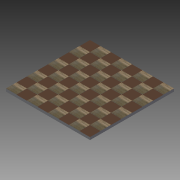
# Autodesk Inventor part: Board 001
Saved by Autodesk Inventor 2015 SP1 (Build 190203100, 203)
## iProperties
Created: 2015-06-07
Part Number: Board 001
Material: Generic
Document SubType Name: Modeling
Designer: Nathan
Density: 1 g/cm^3
Appearance: Default
Author: Nathan
Autodesk Inventor part; units mm, degrees
ref_plane "YZ Plane" through (0, 0, 0) normal (1, 0, 0) x (0, 1, 0)
ref_plane "XZ Plane" through (0, 0, 0) normal (0, 1, 0) x (-1, 0, 0)
ref_plane "XY Plane" through (0, 0, 0) normal (0, 0, 1) x (1, 0, 0)
sketch "Sketch1" plane through (0, 0, 0) normal (0, 1, 0) x (-1, 0, 0)
  line L0 (-180, 180) -> (180, 180)
  line L1 (180, 180) -> (180, -180)
  line L2 (180, -180) -> (-180, -180)
  line L3 (-180, -180) -> (-180, 180)
  line L4 (-180, 180) -> (180, -180) construction
  line L5 (180, 180) -> (-180, -180) construction
  line L6 (180, 180) -> (135, 180)
  line L7 (135, 180) -> (135, 135)
  line L8 (135, 135) -> (180, 135)
  line L9 (180, 135) -> (180, 180)
  line L10 (180, 135) -> (135, 135)
  line L11 (135, 135) -> (135, 90)
  line L12 (135, 90) -> (180, 90)
  line L13 (180, 90) -> (180, 135)
  line L14 (180, 90) -> (135, 90)
  line L15 (135, 90) -> (135, 45)
  line L16 (135, 45) -> (180, 45)
  line L17 (180, 45) -> (180, 90)
  line L18 (180, 45) -> (135, 45)
  line L19 (135, 45) -> (135, 0)
  line L20 (135, 0) -> (180, 0)
  line L21 (180, 0) -> (180, 45)
  line L22 (180, 0) -> (135, 0)
  line L23 (135, 0) -> (135, -45)
  line L24 (135, -45) -> (180, -45)
  line L25 (180, -45) -> (180, 0)
  line L26 (180, -45) -> (135, -45)
  line L27 (135, -45) -> (135, -90)
  line L28 (135, -90) -> (180, -90)
  line L29 (180, -90) -> (180, -45)
  line L30 (180, -90) -> (135, -90)
  line L31 (135, -90) -> (135, -135)
  line L32 (135, -135) -> (180, -135)
  line L33 (180, -135) -> (180, -90)
  line L34 (180, -135) -> (135, -135)
  line L35 (135, -135) -> (135, -180)
  line L36 (135, -180) -> (180, -180)
  line L37 (180, -180) -> (180, -135)
  line L38 (135, 180) -> (90, 180)
  line L39 (90, 180) -> (90, 135)
  line L40 (90, 135) -> (135, 135)
  line L41 (135, 135) -> (135, 180)
  line L42 (135, 135) -> (90, 135)
  line L43 (90, 135) -> (90, 90)
  line L44 (90, 90) -> (135, 90)
  line L45 (135, 90) -> (135, 135)
  line L46 (135, 90) -> (90, 90)
  line L47 (90, 90) -> (90, 45)
  line L48 (90, 45) -> (135, 45)
  line L49 (135, 45) -> (135, 90)
  line L50 (135, 45) -> (90, 45)
  line L51 (90, 45) -> (90, 0)
  line L52 (90, 0) -> (135, 0)
  line L53 (135, 0) -> (135, 45)
  line L54 (135, 0) -> (90, 0)
  line L55 (90, 0) -> (90, -45)
  line L56 (90, -45) -> (135, -45)
  line L57 (135, -45) -> (135, 0)
  line L58 (135, -45) -> (90, -45)
  line L59 (90, -45) -> (90, -90)
  line L60 (90, -90) -> (135, -90)
  line L61 (135, -90) -> (135, -45)
  line L62 (135, -90) -> (90, -90)
  line L63 (90, -90) -> (90, -135)
  line L64 (90, -135) -> (135, -135)
  line L65 (135, -135) -> (135, -90)
  line L66 (135, -135) -> (90, -135)
  line L67 (90, -135) -> (90, -180)
  line L68 (90, -180) -> (135, -180)
  line L69 (135, -180) -> (135, -135)
  line L70 (90, 180) -> (45, 180)
  line L71 (45, 180) -> (45, 135)
  line L72 (45, 135) -> (90, 135)
  line L73 (90, 135) -> (90, 180)
  line L74 (90, 135) -> (45, 135)
  line L75 (45, 135) -> (45, 90)
  line L76 (45, 90) -> (90, 90)
  line L77 (90, 90) -> (90, 135)
  line L78 (90, 90) -> (45, 90)
  line L79 (45, 90) -> (45, 45)
  line L80 (45, 45) -> (90, 45)
  line L81 (90, 45) -> (90, 90)
  line L82 (90, 45) -> (45, 45)
  line L83 (45, 45) -> (45, 0)
  line L84 (45, 0) -> (90, 0)
  line L85 (90, 0) -> (90, 45)
  line L86 (90, 0) -> (45, 0)
  line L87 (45, 0) -> (45, -45)
  line L88 (45, -45) -> (90, -45)
  line L89 (90, -45) -> (90, 0)
  line L90 (90, -45) -> (45, -45)
  line L91 (45, -45) -> (45, -90)
  line L92 (45, -90) -> (90, -90)
  line L93 (90, -90) -> (90, -45)
  line L94 (90, -90) -> (45, -90)
  line L95 (45, -90) -> (45, -135)
  line L96 (45, -135) -> (90, -135)
  line L97 (90, -135) -> (90, -90)
  line L98 (90, -135) -> (45, -135)
  line L99 (45, -135) -> (45, -180)
  line L100 (45, -180) -> (90, -180)
  line L101 (90, -180) -> (90, -135)
  line L102 (45, 180) -> (0, 180)
  line L103 (0, 180) -> (0, 135)
  line L104 (0, 135) -> (45, 135)
  line L105 (45, 135) -> (45, 180)
  line L106 (45, 135) -> (0, 135)
  line L107 (0, 135) -> (0, 90)
  line L108 (0, 90) -> (45, 90)
  line L109 (45, 90) -> (45, 135)
  line L110 (45, 90) -> (0, 90)
  line L111 (0, 90) -> (0, 45)
  line L112 (0, 45) -> (45, 45)
  line L113 (45, 45) -> (45, 90)
  line L114 (45, 45) -> (0, 45)
  line L115 (0, 45) -> (0, 0)
  line L116 (0, 0) -> (45, 0)
  line L117 (45, 0) -> (45, 45)
  line L118 (45, 0) -> (0, 0)
  line L119 (0, 0) -> (0, -45)
  line L120 (0, -45) -> (45, -45)
  line L121 (45, -45) -> (45, 0)
  line L122 (45, -45) -> (0, -45)
  line L123 (0, -45) -> (0, -90)
  line L124 (0, -90) -> (45, -90)
  line L125 (45, -90) -> (45, -45)
  line L126 (45, -90) -> (0, -90)
  line L127 (0, -90) -> (0, -135)
  line L128 (0, -135) -> (45, -135)
  line L129 (45, -135) -> (45, -90)
  line L130 (45, -135) -> (0, -135)
  line L131 (0, -135) -> (0, -180)
  line L132 (0, -180) -> (45, -180)
  line L133 (45, -180) -> (45, -135)
  line L134 (0, 180) -> (-45, 180)
  line L135 (-45, 180) -> (-45, 135)
  line L136 (-45, 135) -> (0, 135)
  line L137 (0, 135) -> (0, 180)
  line L138 (0, 135) -> (-45, 135)
  line L139 (-45, 135) -> (-45, 90)
  line L140 (-45, 90) -> (0, 90)
  line L141 (0, 90) -> (0, 135)
  line L142 (0, 90) -> (-45, 90)
  line L143 (-45, 90) -> (-45, 45)
  line L144 (-45, 45) -> (0, 45)
  line L145 (0, 45) -> (0, 90)
  line L146 (0, 45) -> (-45, 45)
  line L147 (-45, 45) -> (-45, 0)
  line L148 (-45, 0) -> (0, 0)
  line L149 (0, 0) -> (0, 45)
  line L150 (0, 0) -> (-45, 0)
  line L151 (-45, 0) -> (-45, -45)
  line L152 (-45, -45) -> (0, -45)
  line L153 (0, -45) -> (0, 0)
  line L154 (0, -45) -> (-45, -45)
  line L155 (-45, -45) -> (-45, -90)
  line L156 (-45, -90) -> (0, -90)
  line L157 (0, -90) -> (0, -45)
  line L158 (0, -90) -> (-45, -90)
  line L159 (-45, -90) -> (-45, -135)
  line L160 (-45, -135) -> (0, -135)
  line L161 (0, -135) -> (0, -90)
  line L162 (0, -135) -> (-45, -135)
  line L163 (-45, -135) -> (-45, -180)
  line L164 (-45, -180) -> (0, -180)
  line L165 (0, -180) -> (0, -135)
  line L166 (-45, 180) -> (-90, 180)
  line L167 (-90, 180) -> (-90, 135)
  line L168 (-90, 135) -> (-45, 135)
  line L169 (-45, 135) -> (-45, 180)
  line L170 (-45, 135) -> (-90, 135)
  line L171 (-90, 135) -> (-90, 90)
  line L172 (-90, 90) -> (-45, 90)
  line L173 (-45, 90) -> (-45, 135)
  line L174 (-45, 90) -> (-90, 90)
  line L175 (-90, 90) -> (-90, 45)
  line L176 (-90, 45) -> (-45, 45)
  line L177 (-45, 45) -> (-45, 90)
  line L178 (-45, 45) -> (-90, 45)
  line L179 (-90, 45) -> (-90, 0)
  line L180 (-90, 0) -> (-45, 0)
  line L181 (-45, 0) -> (-45, 45)
  line L182 (-45, 0) -> (-90, 0)
  line L183 (-90, 0) -> (-90, -45)
  line L184 (-90, -45) -> (-45, -45)
  line L185 (-45, -45) -> (-45, 0)
  line L186 (-45, -45) -> (-90, -45)
  line L187 (-90, -45) -> (-90, -90)
  line L188 (-90, -90) -> (-45, -90)
  line L189 (-45, -90) -> (-45, -45)
  line L190 (-45, -90) -> (-90, -90)
  line L191 (-90, -90) -> (-90, -135)
  line L192 (-90, -135) -> (-45, -135)
  line L193 (-45, -135) -> (-45, -90)
  line L194 (-45, -135) -> (-90, -135)
  line L195 (-90, -135) -> (-90, -180)
  line L196 (-90, -180) -> (-45, -180)
  line L197 (-45, -180) -> (-45, -135)
  line L198 (-90, 180) -> (-135, 180)
  line L199 (-135, 180) -> (-135, 135)
  line L200 (-135, 135) -> (-90, 135)
  line L201 (-90, 135) -> (-90, 180)
  line L202 (-90, 135) -> (-135, 135)
  line L203 (-135, 135) -> (-135, 90)
  line L204 (-135, 90) -> (-90, 90)
  line L205 (-90, 90) -> (-90, 135)
  line L206 (-90, 90) -> (-135, 90)
  line L207 (-135, 90) -> (-135, 45)
  line L208 (-135, 45) -> (-90, 45)
  line L209 (-90, 45) -> (-90, 90)
  line L210 (-90, 45) -> (-135, 45)
  line L211 (-135, 45) -> (-135, 0)
  line L212 (-135, 0) -> (-90, 0)
  line L213 (-90, 0) -> (-90, 45)
  line L214 (-90, 0) -> (-135, 0)
  line L215 (-135, 0) -> (-135, -45)
  line L216 (-135, -45) -> (-90, -45)
  line L217 (-90, -45) -> (-90, 0)
  line L218 (-90, -45) -> (-135, -45)
  line L219 (-135, -45) -> (-135, -90)
  line L220 (-135, -90) -> (-90, -90)
  line L221 (-90, -90) -> (-90, -45)
  line L222 (-90, -90) -> (-135, -90)
  line L223 (-135, -90) -> (-135, -135)
  line L224 (-135, -135) -> (-90, -135)
  line L225 (-90, -135) -> (-90, -90)
  line L226 (-90, -135) -> (-135, -135)
  line L227 (-135, -135) -> (-135, -180)
  line L228 (-135, -180) -> (-90, -180)
  line L229 (-90, -180) -> (-90, -135)
  line L230 (-135, 180) -> (-180, 180)
  line L231 (-180, 180) -> (-180, 135)
  line L232 (-180, 135) -> (-135, 135)
  line L233 (-135, 135) -> (-135, 180)
  line L234 (-135, 135) -> (-180, 135)
  line L235 (-180, 135) -> (-180, 90)
  line L236 (-180, 90) -> (-135, 90)
  line L237 (-135, 90) -> (-135, 135)
  line L238 (-135, 90) -> (-180, 90)
  line L239 (-180, 90) -> (-180, 45)
  line L240 (-180, 45) -> (-135, 45)
  line L241 (-135, 45) -> (-135, 90)
  line L242 (-135, 45) -> (-180, 45)
  line L243 (-180, 45) -> (-180, 0)
  line L244 (-180, 0) -> (-135, 0)
  line L245 (-135, 0) -> (-135, 45)
  line L246 (-135, 0) -> (-180, 0)
  line L247 (-180, 0) -> (-180, -45)
  line L248 (-180, -45) -> (-135, -45)
  line L249 (-135, -45) -> (-135, 0)
  line L250 (-135, -45) -> (-180, -45)
  line L251 (-180, -45) -> (-180, -90)
  line L252 (-180, -90) -> (-135, -90)
  line L253 (-135, -90) -> (-135, -45)
  line L254 (-135, -90) -> (-180, -90)
  line L255 (-180, -90) -> (-180, -135)
  line L256 (-180, -135) -> (-135, -135)
  line L257 (-135, -135) -> (-135, -90)
  line L258 (-135, -135) -> (-180, -135)
  line L259 (-180, -135) -> (-180, -180)
  line L260 (-180, -180) -> (-135, -180)
  line L261 (-135, -180) -> (-135, -135)
  dimension "d0" = 360
  dimension "d1" = 360
  dimension "d2" = 45
  dimension "d3" = 45
  dimension "d6" = 45
  dimension "d9" = 45
  constraints: 524 end point, 4 parallel, 3 horizontal, 2 midpoint, 2 perpendicular, 1 vertical, 504 other
  measures "d0" distance of L1.end L2.end
  measures "d1" distance of L0.end L1.end
  measures "d2" distance of L8.end L7.end
  measures "d3" distance of L7.end L6.end
  measures "d6" distance of L0.end L10.start
  measures "d9" distance of L0.end L38.start
extrude "Extrusion1" add sketch "Sketch1" against normal blind 11
sketch "Sketch2" plane through (0, 0, 0) normal (0, 1, 0) x (1, 0, 0)
  line L0 (-180, -180) -> (-135, -180)
  line L1 (-135, -180) -> (-135, -135)
  line L2 (-135, -135) -> (-180, -135)
  line L3 (-180, -135) -> (-180, -180)
  line L4 (-180, -90) -> (-135, -90)
  line L5 (-135, -90) -> (-135, -45)
  line L6 (-135, -45) -> (-180, -45)
  line L7 (-180, -45) -> (-180, -90)
  line L8 (-180, 0) -> (-135, 0)
  line L9 (-135, 0) -> (-135, 45)
  line L10 (-135, 45) -> (-180, 45)
  line L11 (-180, 45) -> (-180, 0)
  line L12 (-180, 90) -> (-135, 90)
  line L13 (-135, 90) -> (-135, 135)
  line L14 (-135, 135) -> (-180, 135)
  line L15 (-180, 135) -> (-180, 90)
  line L16 (-90, -180) -> (-45, -180)
  line L17 (-45, -180) -> (-45, -135)
  line L18 (-45, -135) -> (-90, -135)
  line L19 (-90, -135) -> (-90, -180)
  line L20 (-90, -90) -> (-45, -90)
  line L21 (-45, -90) -> (-45, -45)
  line L22 (-45, -45) -> (-90, -45)
  line L23 (-90, -45) -> (-90, -90)
  line L24 (-90, 0) -> (-45, 0)
  line L25 (-45, 0) -> (-45, 45)
  line L26 (-45, 45) -> (-90, 45)
  line L27 (-90, 45) -> (-90, 0)
  line L28 (-90, 90) -> (-45, 90)
  line L29 (-45, 90) -> (-45, 135)
  line L30 (-45, 135) -> (-90, 135)
  line L31 (-90, 135) -> (-90, 90)
  line L32 (0, -180) -> (45, -180)
  line L33 (45, -180) -> (45, -135)
  line L34 (45, -135) -> (0, -135)
  line L35 (0, -135) -> (0, -180)
  line L36 (0, -90) -> (45, -90)
  line L37 (45, -90) -> (45, -45)
  line L38 (45, -45) -> (0, -45)
  line L39 (0, -45) -> (0, -90)
  line L40 (0, 0) -> (45, 0)
  line L41 (45, 0) -> (45, 45)
  line L42 (45, 45) -> (0, 45)
  line L43 (0, 45) -> (0, 0)
  line L44 (0, 90) -> (45, 90)
  line L45 (45, 90) -> (45, 135)
  line L46 (45, 135) -> (0, 135)
  line L47 (0, 135) -> (0, 90)
  line L48 (90, -180) -> (135, -180)
  line L49 (135, -180) -> (135, -135)
  line L50 (135, -135) -> (90, -135)
  line L51 (90, -135) -> (90, -180)
  line L52 (90, -90) -> (135, -90)
  line L53 (135, -90) -> (135, -45)
  line L54 (135, -45) -> (90, -45)
  line L55 (90, -45) -> (90, -90)
  line L56 (90, 0) -> (135, 0)
  line L57 (135, 0) -> (135, 45)
  line L58 (135, 45) -> (90, 45)
  line L59 (90, 45) -> (90, 0)
  line L60 (90, 90) -> (135, 90)
  line L61 (135, 90) -> (135, 135)
  line L62 (135, 135) -> (90, 135)
  line L63 (90, 135) -> (90, 90)
  line L64 (-135, -135) -> (-90, -135)
  line L65 (-90, -135) -> (-90, -90)
  line L66 (-90, -90) -> (-135, -90)
  line L67 (-135, -90) -> (-135, -135)
  line L68 (-135, -45) -> (-90, -45)
  line L69 (-90, -45) -> (-90, 0)
  line L70 (-90, 0) -> (-135, 0)
  line L71 (-135, 0) -> (-135, -45)
  line L72 (-135, 45) -> (-90, 45)
  line L73 (-90, 45) -> (-90, 90)
  line L74 (-90, 90) -> (-135, 90)
  line L75 (-135, 90) -> (-135, 45)
  line L76 (-135, 135) -> (-90, 135)
  line L77 (-90, 135) -> (-90, 180)
  line L78 (-90, 180) -> (-135, 180)
  line L79 (-135, 180) -> (-135, 135)
  line L80 (-45, -135) -> (0, -135)
  line L81 (0, -135) -> (0, -90)
  line L82 (0, -90) -> (-45, -90)
  line L83 (-45, -90) -> (-45, -135)
  line L84 (-45, -45) -> (0, -45)
  line L85 (0, -45) -> (0, 0)
  line L86 (0, 0) -> (-45, 0)
  line L87 (-45, 0) -> (-45, -45)
  line L88 (-45, 45) -> (0, 45)
  line L89 (0, 45) -> (0, 90)
  line L90 (0, 90) -> (-45, 90)
  line L91 (-45, 90) -> (-45, 45)
  line L92 (-45, 135) -> (0, 135)
  line L93 (0, 135) -> (0, 180)
  line L94 (0, 180) -> (-45, 180)
  line L95 (-45, 180) -> (-45, 135)
  line L96 (45, -135) -> (90, -135)
  line L97 (90, -135) -> (90, -90)
  line L98 (90, -90) -> (45, -90)
  line L99 (45, -90) -> (45, -135)
  line L100 (45, -45) -> (90, -45)
  line L101 (90, -45) -> (90, 0)
  line L102 (90, 0) -> (45, 0)
  line L103 (45, 0) -> (45, -45)
  line L104 (45, 45) -> (90, 45)
  line L105 (90, 45) -> (90, 90)
  line L106 (90, 90) -> (45, 90)
  line L107 (45, 90) -> (45, 45)
  line L108 (45, 135) -> (90, 135)
  line L109 (90, 135) -> (90, 180)
  line L110 (90, 180) -> (45, 180)
  line L111 (45, 180) -> (45, 135)
  line L112 (135, -135) -> (180, -135)
  line L113 (180, -135) -> (180, -90)
  line L114 (180, -90) -> (135, -90)
  line L115 (135, -90) -> (135, -135)
  line L116 (135, -45) -> (180, -45)
  line L117 (180, -45) -> (180, 0)
  line L118 (180, 0) -> (135, 0)
  line L119 (135, 0) -> (135, -45)
  line L120 (135, 45) -> (180, 45)
  line L121 (180, 45) -> (180, 90)
  line L122 (180, 90) -> (135, 90)
  line L123 (135, 90) -> (135, 45)
  line L124 (135, 135) -> (180, 135)
  line L125 (180, 135) -> (180, 180)
  line L126 (180, 180) -> (135, 180)
  line L127 (135, 180) -> (135, 135)
  dimension "d14" = 45
  dimension "d15" = 45
  dimension "d18" = 90
  dimension "d21" = 90
  dimension "d28" = 45
  dimension "d29" = 45
  dimension "d30" = 90
  dimension "d31" = 90
  constraints: 256 end point, 4 collinear, 4 horizontal, 4 parallel, 2 perpendicular, 2 vertical, 236 other
  measures "d14" distance of L2.end L1.end
  measures "d15" distance of L1.end L0.end
  measures "d18" distance of L1.end L5.end
  measures "d21" distance of L1.end L17.end
  measures "d28" distance of L66.end L65.end
  measures "d29" distance of L65.end L64.end
  measures "d30" distance of L65.end L69.end
  measures "d31" distance of L65.end L81.end
extrude "Extrusion2" add sketch "Sketch2" along normal blind 0.5 contours L3 L2 L1 L0 | L127 L126 L125 L124 | L67 L66 L65 L64 | L18 L17 L16 L19 | L4 L7 L6 L5 | L83 L82 L81 L80 | L23 L22 L21 L20 | L71 L70 L69 L68 | L34 L33 L32 L35 | L8 L11 L10 L9 | L99 L98 L97 L96 | L39 L38 L37 L36 | L87 L86 L85 L84 | L27 L26 L25 L24 | L75 L74 L73 L72 | L50 L49 L48 L51 | L12 L15 L14 L13 | L115 L114 L113 L112 | L55 L54 L53 L52 | L103 L102 L101 L100 | L43 L42 L41 L40 | L91 L90 L89 L88 | L31 L30 L29 L28 | L79 L78 L77 L76 | L119 L118 L117 L116 | L59 L58 L57 L56 | L107 L106 L105 L104 | L47 L46 L45 L44 | L95 L94 L93 L92 | L123 L122 L121 L120 | L63 L62 L61 L60 | L111 L110 L109 L108
body "Solid1"
